Motor Bracket_v11 (Autodesk Fusion 360 design; units mm, degrees)
Autodesk Fusion 360 part; units mm, degrees
note: some values were not read from the file. Set by a fixed rule: which sketch regions a step uses.
sketch "Sketch1" plane through (0, 0, 0) normal (0, 0, 1) x (1, 0, 0)
  circle A0 centre (0, 0) radius 62.75
  circle A1 centre (0, 0) radius 60
  dimension "d1" = 125.5
  dimension "d5" = 120
  constraint coincident A0.centre A1.centre
  measures "d1" diameter of A0
  measures "d5" diameter of A1
extrude "Extrude2" add sketch "Sketch1" along normal blind 5 contours A0 | A1
extrude "Extrude3" add sketch "Sketch1" along normal blind 48.8
sketch "Attachment Point" plane through (0, 0, 48.8) normal (0, 0, 1) x (-1, 0, 0)
  circle A0 centre (0, 0) radius 60
  circle A1 centre (0, 0) radius 62.75
  circle A2 centre (0, 0) radius 57.5
  circle A3 centre (0, 0) radius 65
  dimension "d14" = 115
  dimension "d15" = 130
  constraint coincident A0.centre A1.centre
  constraint concentric A2 A3
  measures "d14" diameter of A2
  measures "d15" diameter of A3
extrude "Extrude4" add sketch "Attachment Point" along normal blind 5 contours A0 | A1 | A3
fillet "Fillet1" radius 2.5 2 edges at (53.6088, -20.7929, 48.8) (60.6013, 23.505, 48.8)
fillet "Fillet2" radius 5 1 edges at (-55.9396, -21.6969, 5)
sketch "CutOuts" plane through (0, 0, 0) normal (0, 0, 1) x (1, 0, 0)
  circle A0 centre (0, -60) radius 12.5
  circle A1 centre (0, 0) radius 60
  circle A2 centre (0, 0) radius 20
  spline S0 degree 2 poles (12.432, -58.6979) (0, -7.3157) (-12.432, -58.6979) knots 0 0 0 8.098463 8.098463 8.098463 weights 1 3 1
  dimension "d20" = 25
  dimension "d21" = 40
  constraint coincident A0.centre A1
  constraint concentric A1 A2
  constraint coincident A0 S0.end
  constraint coincident A1 S0.end
  constraint coincident A0 S0.start
  constraint coincident A1 S0.start
  measures "d20" diameter of A0
  measures "d21" diameter of A2
extrude "Extrude5" cut sketch "CutOuts" along normal blind 48.8 contours A0 A1 | A0 A1 S0 | A0 S0 picked at (0, -55.7366) picked at (0.2989, -34.7266)
pattern_circular "C-Pattern1" count 6 over 360 about axis through (0, 0, 1.75) along (0, 0, 1) of "Extrude5"
sketch "Bracket Mount Holes" plane through (0, 0, 48.8) normal (0, 0, -1) x (1, 0, 0)
  arc A0 (12.4083, 61.5109) -> (-12.4083, 61.5109) centre (0, 0) ccw
  arc A1 (-12.4083, 61.5109) -> (-12.432, 58.6979) centre (0, 60) ccw
  arc A2 (12.432, 58.6979) -> (-12.432, 58.6979) centre (0, 0) ccw
  arc A3 (12.432, 58.6979) -> (12.4083, 61.5109) centre (0, 60) ccw
  circle A4 centre (0, 61.375) radius 1.5
  line L0 (0, 61.375) -> (0, 60) construction
  dimension "d30" = 3
  dimension "d31" = 1.375
  constraint coincident A4.centre L0.start
  constraint coincident A1.centre A3.centre
  constraint vertical L0
  measures "d30" diameter of A4
  measures "d31" distance of A4.centre A1.centre
extrude "Extrude6" cut sketch "Bracket Mount Holes" against normal blind 8 contours A0 A2 A4 | A0 A4 | A2 A4
pattern_circular "C-Pattern2" count 6 over 360 about axis through (0, 0, 1.75) along (0, 0, 1) of "Extrude6"
sketch "Encoder Holes" plane through (0, 0, 0) normal (0, 0, -1) x (1, 0, 0)
  arc A0 (-44.6179, 40.1154) -> (-47.0659, 41.5014) centre (-51.9615, 30) ccw
  spline S0 degree 2 poles (-44.6179, 40.1154) (-43.3703, 38.9273) (-42.2032, 37.8118) knots 0 0 0 0.089929 0.089929 0.089929 weights 1 1.022209 1.043925
  spline S1 degree 2 poles (-42.2032, 37.8118) (-6.6662, 3.8487) (-53.8476, 17.6431) knots 0.089929 0.089929 0.089929 8.008534 8.008534 8.008534 weights 1.043925 2.956075 1.043925
  spline S2 degree 2 poles (-53.8476, 17.6431) (-55.3971, 18.0961) (-57.0499, 18.5825) knots 8.008534 8.008534 8.008534 8.098463 8.098463 8.098463 weights 1.043925 1.022209 1
  arc A1 (-59.4742, 20.0095) -> (-57.0499, 18.5825) centre (-51.9615, 30) ccw
  arc A2 (-59.4742, 20.0095) -> (-59.4742, -20.0095) centre (0, 0) ccw
  arc A3 (-57.0499, -18.5825) -> (-59.4742, -20.0095) centre (-51.9615, -30) ccw
  spline S3 degree 2 poles (-57.0499, -18.5825) (-55.3971, -18.0961) (-53.8476, -17.6431) knots 0 0 0 0.089929 0.089929 0.089929 weights 1 1.022209 1.043925
  spline S4 degree 2 poles (-53.8476, -17.6431) (-6.6662, -3.8487) (-42.2032, -37.8118) knots 0.089929 0.089929 0.089929 8.008534 8.008534 8.008534 weights 1.043925 2.956075 1.043925
  spline S5 degree 2 poles (-42.2032, -37.8118) (-43.3703, -38.9273) (-44.6179, -40.1154) knots 8.008534 8.008534 8.008534 8.098463 8.098463 8.098463 weights 1.043925 1.022209 1
  arc A4 (-47.0659, -41.5014) -> (-44.6179, -40.1154) centre (-51.9615, -30) ccw
  arc A5 (-47.0659, -41.5014) -> (-12.4083, -61.5109) centre (0, 0) ccw
  arc A6 (-12.432, -58.6979) -> (-12.4083, -61.5109) centre (0, -60) ccw
  spline S6 degree 2 poles (-12.432, -58.6979) (-12.0268, -57.0234) (-11.6444, -55.455) knots 0 0 0 0.089929 0.089929 0.089929 weights 1 1.022209 1.043925
  spline S7 degree 2 poles (-11.6444, -55.455) (0, -7.6975) (11.6444, -55.455) knots 0.089929 0.089929 0.089929 8.008534 8.008534 8.008534 weights 1.043925 2.956075 1.043925
  spline S8 degree 2 poles (11.6444, -55.455) (12.0268, -57.0234) (12.432, -58.6979) knots 8.008534 8.008534 8.008534 8.098463 8.098463 8.098463 weights 1.043925 1.022209 1
  arc A7 (12.4083, -61.5109) -> (12.432, -58.6979) centre (0, -60) ccw
  arc A8 (12.4083, -61.5109) -> (47.0659, -41.5014) centre (0, 0) ccw
  arc A9 (44.6179, -40.1154) -> (47.0659, -41.5014) centre (51.9615, -30) ccw
  spline S9 degree 2 poles (44.6179, -40.1154) (43.3703, -38.9273) (42.2032, -37.8118) knots 0 0 0 0.089929 0.089929 0.089929 weights 1 1.022209 1.043925
  spline S10 degree 2 poles (42.2032, -37.8118) (6.6662, -3.8487) (53.8476, -17.6431) knots 0.089929 0.089929 0.089929 8.008534 8.008534 8.008534 weights 1.043925 2.956075 1.043925
  spline S11 degree 2 poles (53.8476, -17.6431) (55.3971, -18.0961) (57.0499, -18.5825) knots 8.008534 8.008534 8.008534 8.098463 8.098463 8.098463 weights 1.043925 1.022209 1
  arc A10 (59.4742, -20.0095) -> (57.0499, -18.5825) centre (51.9615, -30) ccw
  arc A11 (59.4742, -20.0095) -> (59.4742, 20.0095) centre (0, 0) ccw
  arc A12 (57.0499, 18.5825) -> (59.4742, 20.0095) centre (51.9615, 30) ccw
  spline S12 degree 2 poles (57.0499, 18.5825) (55.3971, 18.0961) (53.8476, 17.6431) knots 0 0 0 0.089929 0.089929 0.089929 weights 1 1.022209 1.043925
  spline S13 degree 2 poles (53.8476, 17.6431) (6.6662, 3.8487) (42.2032, 37.8118) knots 0.089929 0.089929 0.089929 8.008534 8.008534 8.008534 weights 1.043925 2.956075 1.043925
  spline S14 degree 2 poles (42.2032, 37.8118) (43.3703, 38.9273) (44.6179, 40.1154) knots 8.008534 8.008534 8.008534 8.098463 8.098463 8.098463 weights 1.043925 1.022209 1
  arc A13 (47.0659, 41.5014) -> (44.6179, 40.1154) centre (51.9615, 30) ccw
  arc A14 (47.0659, 41.5014) -> (12.4083, 61.5109) centre (0, 0) ccw
  arc A15 (12.432, 58.6979) -> (12.4083, 61.5109) centre (0, 60) ccw
  spline S15 degree 2 poles (12.432, 58.6979) (12.0268, 57.0234) (11.6444, 55.455) knots 0 0 0 0.089929 0.089929 0.089929 weights 1 1.022209 1.043925
  spline S16 degree 2 poles (11.6444, 55.455) (0, 7.6975) (-11.6444, 55.455) knots 0.089929 0.089929 0.089929 8.008534 8.008534 8.008534 weights 1.043925 2.956075 1.043925
  spline S17 degree 2 poles (-11.6444, 55.455) (-12.0268, 57.0234) (-12.432, 58.6979) knots 8.008534 8.008534 8.008534 8.098463 8.098463 8.098463 weights 1.043925 1.022209 1
  arc A16 (-12.4083, 61.5109) -> (-12.432, 58.6979) centre (0, 60) ccw
  arc A17 (-12.4083, 61.5109) -> (-47.0659, 41.5014) centre (0, 0) ccw
  line L0 (-5.5, 9) -> (5.5, 9) construction
  line L1 (5.5, 9) -> (5.5, -9) construction
  line L2 (5.5, -9) -> (-5.5, -9) construction
  line L3 (-5.5, -9) -> (-5.5, 9) construction
  line L4 (-5.5, 9) -> (5.5, -9) construction
  line L5 (5.5, 9) -> (-5.5, -9) construction
  circle A18 centre (5.5, -9) radius 1
  circle A19 centre (-5.5, -9) radius 1
  circle A20 centre (5.5, 9) radius 1
  circle A21 centre (-5.5, 9) radius 1
  circle A22 centre (0, 0) radius 6.5
  dimension "d36" = 11
  dimension "d37" = 18
  dimension "d39" = 2
  dimension "d40" = 2
  dimension "d41" = 2
  dimension "d42" = 2
  dimension "d43" = 13
  constraint horizontal L0
  constraint perpendicular L0 L1
  constraint parallel L0 L2
  constraint parallel L1 L3
  constraint coincident L4 A2.centre
  constraint coincident L5 A2.centre
  constraint coincident A2.centre A5.centre
  constraint coincident L1.end L2.start
  constraint coincident L2.end L3.start
  constraint coincident L0.end L1.start
  constraint coincident L0.start L3.end
  measures "d36" distance of L1.end L2.end
  measures "d37" distance of L0.end L1.end
  measures "d39" diameter of A18
  measures "d40" diameter of A19
  measures "d41" diameter of A20
  measures "d42" diameter of A21
  measures "d43" diameter of A22
extrude "Extrude7" [suppressed]
sketch "MotorScrews" plane through (0, 0, 0) normal (0, 0, -1) x (1, 0, 0)
  circle A0 centre (0, 0) radius 6.5
  circle A1 centre (-5.5, -9) radius 1
  circle A2 centre (-5.5, 9) radius 1
  circle A3 centre (5.5, -9) radius 1
  circle A4 centre (5.5, 9) radius 1
  arc A5 (-44.6179, 40.1154) -> (-47.0659, 41.5014) centre (-51.9615, 30) ccw
  spline S0 degree 2 poles (-44.6179, 40.1154) (-43.3703, 38.9273) (-42.2032, 37.8118) knots 0 0 0 0.089929 0.089929 0.089929 weights 1 1.022209 1.043925
  spline S1 degree 2 poles (-42.2032, 37.8118) (-6.6662, 3.8487) (-53.8476, 17.6431) knots 0.089929 0.089929 0.089929 8.008534 8.008534 8.008534 weights 1.043925 2.956075 1.043925
  spline S2 degree 2 poles (-53.8476, 17.6431) (-55.3971, 18.0961) (-57.0499, 18.5825) knots 8.008534 8.008534 8.008534 8.098463 8.098463 8.098463 weights 1.043925 1.022209 1
  arc A6 (-59.4742, 20.0095) -> (-57.0499, 18.5825) centre (-51.9615, 30) ccw
  arc A7 (-59.4742, 20.0095) -> (-59.4742, -20.0095) centre (0, 0) ccw
  arc A8 (-57.0499, -18.5825) -> (-59.4742, -20.0095) centre (-51.9615, -30) ccw
  spline S3 degree 2 poles (-57.0499, -18.5825) (-55.3971, -18.0961) (-53.8476, -17.6431) knots 0 0 0 0.089929 0.089929 0.089929 weights 1 1.022209 1.043925
  spline S4 degree 2 poles (-53.8476, -17.6431) (-6.6662, -3.8487) (-42.2032, -37.8118) knots 0.089929 0.089929 0.089929 8.008534 8.008534 8.008534 weights 1.043925 2.956075 1.043925
  spline S5 degree 2 poles (-42.2032, -37.8118) (-43.3703, -38.9273) (-44.6179, -40.1154) knots 8.008534 8.008534 8.008534 8.098463 8.098463 8.098463 weights 1.043925 1.022209 1
  arc A9 (-47.0659, -41.5014) -> (-44.6179, -40.1154) centre (-51.9615, -30) ccw
  arc A10 (-47.0659, -41.5014) -> (-12.4083, -61.5109) centre (0, 0) ccw
  arc A11 (-12.432, -58.6979) -> (-12.4083, -61.5109) centre (0, -60) ccw
  spline S6 degree 2 poles (-12.432, -58.6979) (-12.0268, -57.0234) (-11.6444, -55.455) knots 0 0 0 0.089929 0.089929 0.089929 weights 1 1.022209 1.043925
  spline S7 degree 2 poles (-11.6444, -55.455) (0, -7.6975) (11.6444, -55.455) knots 0.089929 0.089929 0.089929 8.008534 8.008534 8.008534 weights 1.043925 2.956075 1.043925
  spline S8 degree 2 poles (11.6444, -55.455) (12.0268, -57.0234) (12.432, -58.6979) knots 8.008534 8.008534 8.008534 8.098463 8.098463 8.098463 weights 1.043925 1.022209 1
  arc A12 (12.4083, -61.5109) -> (12.432, -58.6979) centre (0, -60) ccw
  arc A13 (12.4083, -61.5109) -> (47.0659, -41.5014) centre (0, 0) ccw
  arc A14 (44.6179, -40.1154) -> (47.0659, -41.5014) centre (51.9615, -30) ccw
  spline S9 degree 2 poles (44.6179, -40.1154) (43.3703, -38.9273) (42.2032, -37.8118) knots 0 0 0 0.089929 0.089929 0.089929 weights 1 1.022209 1.043925
  spline S10 degree 2 poles (42.2032, -37.8118) (6.6662, -3.8487) (53.8476, -17.6431) knots 0.089929 0.089929 0.089929 8.008534 8.008534 8.008534 weights 1.043925 2.956075 1.043925
  spline S11 degree 2 poles (53.8476, -17.6431) (55.3971, -18.0961) (57.0499, -18.5825) knots 8.008534 8.008534 8.008534 8.098463 8.098463 8.098463 weights 1.043925 1.022209 1
  arc A15 (59.4742, -20.0095) -> (57.0499, -18.5825) centre (51.9615, -30) ccw
  arc A16 (59.4742, -20.0095) -> (59.4742, 20.0095) centre (0, 0) ccw
  arc A17 (57.0499, 18.5825) -> (59.4742, 20.0095) centre (51.9615, 30) ccw
  spline S12 degree 2 poles (57.0499, 18.5825) (55.3971, 18.0961) (53.8476, 17.6431) knots 0 0 0 0.089929 0.089929 0.089929 weights 1 1.022209 1.043925
  spline S13 degree 2 poles (53.8476, 17.6431) (6.6662, 3.8487) (42.2032, 37.8118) knots 0.089929 0.089929 0.089929 8.008534 8.008534 8.008534 weights 1.043925 2.956075 1.043925
  spline S14 degree 2 poles (42.2032, 37.8118) (43.3703, 38.9273) (44.6179, 40.1154) knots 8.008534 8.008534 8.008534 8.098463 8.098463 8.098463 weights 1.043925 1.022209 1
  arc A18 (47.0659, 41.5014) -> (44.6179, 40.1154) centre (51.9615, 30) ccw
  arc A19 (47.0659, 41.5014) -> (12.4083, 61.5109) centre (0, 0) ccw
  arc A20 (12.432, 58.6979) -> (12.4083, 61.5109) centre (0, 60) ccw
  spline S15 degree 2 poles (12.432, 58.6979) (12.0268, 57.0234) (11.6444, 55.455) knots 0 0 0 0.089929 0.089929 0.089929 weights 1 1.022209 1.043925
  spline S16 degree 2 poles (11.6444, 55.455) (0, 7.6975) (-11.6444, 55.455) knots 0.089929 0.089929 0.089929 8.008534 8.008534 8.008534 weights 1.043925 2.956075 1.043925
  spline S17 degree 2 poles (-11.6444, 55.455) (-12.0268, 57.0234) (-12.432, 58.6979) knots 8.008534 8.008534 8.008534 8.098463 8.098463 8.098463 weights 1.043925 1.022209 1
  arc A21 (-12.4083, 61.5109) -> (-12.432, 58.6979) centre (0, 60) ccw
  arc A22 (-12.4083, 61.5109) -> (-47.0659, 41.5014) centre (0, 0) ccw
  circle A23 centre (0, 0) radius 12.75 construction
  circle A24 centre (0, -12.75) radius 1.5
  circle A25 centre (0, -12.75) radius 2.5
  dimension "d49" = 25.5
  dimension "d50" = 3
  dimension "d51" = 5
  constraint coincident A0.centre A7.centre
  constraint coincident A23 A24.centre
  constraint concentric A24 A25
  measures "d49" diameter of A23
  measures "d50" diameter of A24
  measures "d51" diameter of A25
extrude "Extrude8" [suppressed]
extrude "Extrude9" [suppressed]
pattern_circular "C-Pattern3" [suppressed]
sketch "Sketch8" plane through (0, 0, 0) normal (0, 0, -1) x (1, 0, 0)
  circle A0 centre (12.75, 0) radius 2.5
  circle A1 centre (0, 12.75) radius 2.5
  circle A2 centre (-12.75, 0) radius 2.5
  circle A3 centre (0, -12.75) radius 2.5
  circle A4 centre (0, 0) radius 6.5
  circle A5 centre (-5.5, -9) radius 1
  circle A6 centre (-5.5, 9) radius 1
  circle A7 centre (5.5, -9) radius 1
  circle A8 centre (5.5, 9) radius 1
  arc A9 (-44.6179, 40.1154) -> (-47.0659, 41.5014) centre (-51.9615, 30) ccw
  spline S0 degree 2 poles (-44.6179, 40.1154) (-43.3703, 38.9273) (-42.2032, 37.8118) knots 0 0 0 0.089929 0.089929 0.089929 weights 1 1.022209 1.043925
  spline S1 degree 2 poles (-42.2032, 37.8118) (-6.6662, 3.8487) (-53.8476, 17.6431) knots 0.089929 0.089929 0.089929 8.008534 8.008534 8.008534 weights 1.043925 2.956075 1.043925
  spline S2 degree 2 poles (-53.8476, 17.6431) (-55.3971, 18.0961) (-57.0499, 18.5825) knots 8.008534 8.008534 8.008534 8.098463 8.098463 8.098463 weights 1.043925 1.022209 1
  arc A10 (-59.4742, 20.0095) -> (-57.0499, 18.5825) centre (-51.9615, 30) ccw
  arc A11 (-59.4742, 20.0095) -> (-59.4742, -20.0095) centre (0, 0) ccw
  arc A12 (-57.0499, -18.5825) -> (-59.4742, -20.0095) centre (-51.9615, -30) ccw
  spline S3 degree 2 poles (-57.0499, -18.5825) (-55.3971, -18.0961) (-53.8476, -17.6431) knots 0 0 0 0.089929 0.089929 0.089929 weights 1 1.022209 1.043925
  spline S4 degree 2 poles (-53.8476, -17.6431) (-6.6662, -3.8487) (-42.2032, -37.8118) knots 0.089929 0.089929 0.089929 8.008534 8.008534 8.008534 weights 1.043925 2.956075 1.043925
  spline S5 degree 2 poles (-42.2032, -37.8118) (-43.3703, -38.9273) (-44.6179, -40.1154) knots 8.008534 8.008534 8.008534 8.098463 8.098463 8.098463 weights 1.043925 1.022209 1
  arc A13 (-47.0659, -41.5014) -> (-44.6179, -40.1154) centre (-51.9615, -30) ccw
  arc A14 (-47.0659, -41.5014) -> (-12.4083, -61.5109) centre (0, 0) ccw
  arc A15 (-12.432, -58.6979) -> (-12.4083, -61.5109) centre (0, -60) ccw
  spline S6 degree 2 poles (-12.432, -58.6979) (-12.0268, -57.0234) (-11.6444, -55.455) knots 0 0 0 0.089929 0.089929 0.089929 weights 1 1.022209 1.043925
  spline S7 degree 2 poles (-11.6444, -55.455) (0, -7.6975) (11.6444, -55.455) knots 0.089929 0.089929 0.089929 8.008534 8.008534 8.008534 weights 1.043925 2.956075 1.043925
  spline S8 degree 2 poles (11.6444, -55.455) (12.0268, -57.0234) (12.432, -58.6979) knots 8.008534 8.008534 8.008534 8.098463 8.098463 8.098463 weights 1.043925 1.022209 1
  arc A16 (12.4083, -61.5109) -> (12.432, -58.6979) centre (0, -60) ccw
  arc A17 (12.4083, -61.5109) -> (47.0659, -41.5014) centre (0, 0) ccw
  arc A18 (44.6179, -40.1154) -> (47.0659, -41.5014) centre (51.9615, -30) ccw
  spline S9 degree 2 poles (44.6179, -40.1154) (43.3703, -38.9273) (42.2032, -37.8118) knots 0 0 0 0.089929 0.089929 0.089929 weights 1 1.022209 1.043925
  spline S10 degree 2 poles (42.2032, -37.8118) (6.6662, -3.8487) (53.8476, -17.6431) knots 0.089929 0.089929 0.089929 8.008534 8.008534 8.008534 weights 1.043925 2.956075 1.043925
  spline S11 degree 2 poles (53.8476, -17.6431) (55.3971, -18.0961) (57.0499, -18.5825) knots 8.008534 8.008534 8.008534 8.098463 8.098463 8.098463 weights 1.043925 1.022209 1
  arc A19 (59.4742, -20.0095) -> (57.0499, -18.5825) centre (51.9615, -30) ccw
  arc A20 (59.4742, -20.0095) -> (59.4742, 20.0095) centre (0, 0) ccw
  arc A21 (57.0499, 18.5825) -> (59.4742, 20.0095) centre (51.9615, 30) ccw
  spline S12 degree 2 poles (57.0499, 18.5825) (55.3971, 18.0961) (53.8476, 17.6431) knots 0 0 0 0.089929 0.089929 0.089929 weights 1 1.022209 1.043925
  spline S13 degree 2 poles (53.8476, 17.6431) (6.6662, 3.8487) (42.2032, 37.8118) knots 0.089929 0.089929 0.089929 8.008534 8.008534 8.008534 weights 1.043925 2.956075 1.043925
  spline S14 degree 2 poles (42.2032, 37.8118) (43.3703, 38.9273) (44.6179, 40.1154) knots 8.008534 8.008534 8.008534 8.098463 8.098463 8.098463 weights 1.043925 1.022209 1
  arc A22 (47.0659, 41.5014) -> (44.6179, 40.1154) centre (51.9615, 30) ccw
  arc A23 (47.0659, 41.5014) -> (12.4083, 61.5109) centre (0, 0) ccw
  arc A24 (12.432, 58.6979) -> (12.4083, 61.5109) centre (0, 60) ccw
  spline S15 degree 2 poles (12.432, 58.6979) (12.0268, 57.0234) (11.6444, 55.455) knots 0 0 0 0.089929 0.089929 0.089929 weights 1 1.022209 1.043925
  spline S16 degree 2 poles (11.6444, 55.455) (0, 7.6975) (-11.6444, 55.455) knots 0.089929 0.089929 0.089929 8.008534 8.008534 8.008534 weights 1.043925 2.956075 1.043925
  spline S17 degree 2 poles (-11.6444, 55.455) (-12.0268, 57.0234) (-12.432, 58.6979) knots 8.008534 8.008534 8.008534 8.098463 8.098463 8.098463 weights 1.043925 1.022209 1
  arc A25 (-12.4083, 61.5109) -> (-12.432, 58.6979) centre (0, 60) ccw
  arc A26 (-12.4083, 61.5109) -> (-47.0659, 41.5014) centre (0, 0) ccw
ref_plane "WorkPlane1" through (0, 0, -8) normal (0, 0, -1) x (1, 0, 0)
sketch "Sketch10" plane through (0, 0, -8) normal (0, 0, -1) x (1, 0, 0)
  circle A0 centre (0, 0) radius 20
  circle A1 centre (0, 0) radius 16 construction
  circle A2 centre (14.3945, 6.9856) radius 2
  line L0 (20, 0) -> (2.5, 0)
  circle A3 centre (14.3945, -6.9856) radius 2
  line L1 (0, -2.5) -> (0, -20)
  circle A4 centre (-14.3945, -6.9856) radius 2
  circle A5 centre (-14.3945, 6.9856) radius 2
  circle A6 centre (14.3945, 6.9856) radius 1
  circle A7 centre (14.3945, -6.9856) radius 1
  circle A8 centre (-14.3945, -6.9856) radius 1
  circle A9 centre (-14.3945, 6.9856) radius 1
  dimension "d62" = 40
  dimension "d63" = 32
  dimension "d64" = 4
  dimension "d65" = 2
  dimension "d66" = 2
  dimension "d67" = 2
  dimension "d68" = 2
  constraint coincident A0.centre A1.centre
  constraint coincident A1 A2.centre
  constraint symmetric A2 L0 A3
  constraint symmetric A2 L1 A5
  constraint symmetric A3 L1 A4
  constraint concentric A2 A6
  constraint concentric A3 A7
  constraint concentric A4 A8
  constraint concentric A5 A9
  measures "d62" diameter of A0
  measures "d63" diameter of A1
  measures "d64" diameter of A2
  measures "d65" diameter of A6
  measures "d66" diameter of A7
  measures "d67" diameter of A8
  measures "d68" diameter of A9
extrude "Extrude10" [suppressed]
extrude "Extrude11" [suppressed]
extrude "Extrude12" [suppressed]
fillet "Fillet3" [suppressed]
fillet "Fillet4" [suppressed]
equation "sdf = BracketDepth"
equation "sdff = OffsetHieght"
equation "OffsetHieght = MotorHeight + BracketDepth + CouplingLenght"
equation "MotorHeight = 33.8 mm"
equation "BracketDepth = 5 mm"
equation "CouplingLenght = 10 mm"
equation "d23 = OffsetHieght"
equation "BracketScrewDia = 2 mm"
equation "d37 = EncoderBracketCoverHolePattern"
equation "EncoderScrew = 2 mm"
equation "d39 = EncoderScrew"
equation "d40 = EncoderScrew"
equation "d41 = EncoderScrew"
equation "d42 = EncoderScrew"
equation "MotorMountDia = 25.5 mm"
equation "MotorMountScrewDia = 3 mm"
equation "MotorMountScrewHead = 5 mm"
equation "d49 = MotorMountDia"
equation "d50 = MotorMountScrewDia"
equation "d51 = MotorMountScrewHead"
equation "d54 = -BracketDepth"
equation "EncoderBracketCoverHolePattern = 18 mm"
